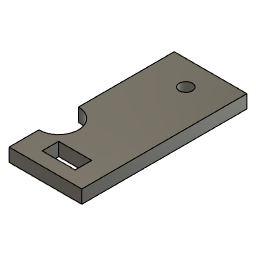
Test1 v2 (Autodesk Fusion 360 design; units mm, degrees)
Autodesk Fusion 360 part; units mm, degrees
sketch "草图1" plane through (0, 0, 0) normal (0, 1, 0) x (1, 0, 0)
  circle A0 centre (0, 0) radius 6
  line L0 (6, -6) -> (16, -6)
  line L1 (16, -6) -> (16, -11)
  line L2 (16, -11) -> (6, -11)
  line L3 (6, -11) -> (6, -6)
  line L4 (11, -6) -> (11, 27.5)
  circle A1 centre (11, 27.5) radius 2
  line L5 (0, 0) -> (0, 35)
  line L6 (0, 35) -> (22, 35)
  line L7 (22, 35) -> (22, -15)
  line L8 (22, -15) -> (0, -15)
  line L9 (0, -15) -> (0, 0)
  dimension "d1" = 12
  dimension "d3" = 10
  dimension "d4" = 5
  constraint coincident A0.centre L5.start
  constraint perpendicular L0 L1
  constraint perpendicular L1 L2
  constraint perpendicular L0 L3
  constraint midpoint L0 L4.start
  constraint coincident L4.end A1.centre
  constraint perpendicular L5 L6
  constraint perpendicular L7 L8
  measures "d1" diameter of A0
  measures "d3" distance of L0.start L0.end
  measures "d4" distance of L0.end L1.end
extrude "拉伸1" add sketch "草图1" against normal blind 4 contours A0 L5 L6 L7 L8 L9
